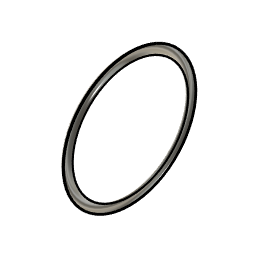
front_rim_eng_model (Autodesk Fusion 360 design; units mm, degrees)
Autodesk Fusion 360 part; units mm, degrees
sketch "Sketch1" plane through (0, 0, 0) normal (0, 1, 0) x (1, 0, 0)
  line L0 (0, 0) -> (0, -260) construction
  line L1 (0, -260) -> (0, -293.0516) construction
  arc A0 (0, -240) -> (-5.1764, -279.3185) centre (0, -260) ccw
  arc A1 (0, -243) -> (-4.3999, -276.4207) centre (0, -260) ccw
  line L2 (0, -260) -> (-1.2338, -260) construction
  line L3 (0, -260) -> (0, -261.669)
  line L4 (-4.3999, -276.4207) -> (-4.0117, -274.9719)
  line L5 (-4.0117, -274.9719) -> (-1.1139, -275.7483)
  line L6 (-1.1139, -275.7483) -> (-1.8904, -278.6461)
  line L7 (-1.8904, -278.6461) -> (-4.7882, -277.8696)
  line L8 (-5.1764, -279.3185) -> (-4.7882, -277.8696)
  line L9 (0, -260) -> (-4.3999, -276.4207) construction
  line L10 (-4.7882, -277.8696) -> (-7.1562, -286.7073) construction
  line L11 (0, -240) -> (0, -243)
  dimension "d2" = 40
  dimension "d3" = 34
  dimension "d4" = 15
  dimension "d6" = 3
  dimension "d7" = 3
  dimension "d8" = 3
  dimension "d10" = 240
  dimension "d11" = 260
  constraint coincident L0.start origin
  constraint vertical L0
  constraint coincident L0.end L1.start
  constraint concentric A0 A1
  constraint parallel L0 L1
  constraint coincident L0 A0.start
  constraint coincident L0 A1.start
  constraint perpendicular L1 L2
  constraint coincident L1 L3.end
  constraint perpendicular L2 L3
  constraint coincident A0.end L9
  constraint coincident L7.end L9
  constraint parallel L4 L9
  constraint perpendicular L5 L9
  constraint perpendicular L5 L6
  constraint collinear L9 L10
  measures "d2" diameter of A0
  measures "d3" diameter of A1
  measures "d4" angle of L1 L9
  measures "d6" distance of L7.end L4.end
  measures "d7" distance of L4.end L5.end
  measures "d8" distance of L5.end L6.end
  measures "d10" distance of L0.start A0.start
  measures "d11" distance of L0.start L0.end
revolve "Revolve1" add sketch "Sketch1" angle 360 about axis through (1.75, 0, 0) along (1, 0, 0)
equation "d3 = ( 17 * 2 ) * 1 mm"
